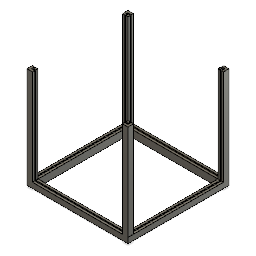
Bofy-top (Autodesk Fusion 360 design; units mm, degrees)
Autodesk Fusion 360 part; units mm, degrees
sketch "Sketch10" plane through (0, 0, 0) normal (0, 1, 0) x (1, 0, 0)
  line L0 (-70, -70) -> (100, -70)
  line L1 (100, -70) -> (100, 100)
  line L2 (100, 100) -> (-70, 100)
  line L3 (-70, 100) -> (-70, -70)
  dimension "d21" = 170
  dimension "d22" = 170
  constraint horizontal L0
  constraint vertical L1
  constraint horizontal L2
  constraint vertical L3
  measures "d21" distance of L0.start L0.end
  measures "d22" distance of L0.start L2.end
extrude "Extrude8" add sketch "Sketch10" along normal blind 8 makes body 1
sketch "Sketch11" plane through (0, 8, 0) normal (0, 1, 0) x (-1, 0, 0)
  line L0 (70, -100) -> (70, 70)
  line L1 (70, 70) -> (-100, 70)
  line L2 (-100, 70) -> (-100, -100)
  line L3 (-100, -100) -> (70, -100)
  line L4 (65, -95) -> (-95, -95)
  line L5 (-95, -95) -> (-95, 65)
  line L6 (-95, 65) -> (65, 65)
  line L7 (65, 65) -> (65, -95)
  constraint horizontal L4
  constraint vertical L5
  constraint horizontal L6
  constraint vertical L7
extrude "Extrude9" cut sketch "Sketch11" against normal blind 8 contours L4 L5 L6 L7 bodies 1
sketch "Sketch12" plane through (0, 8, 0) normal (0, 1, 0) x (-1, 0, 0)
  line L0 (-95, -95) -> (-95, 65)
  line L1 (-95, 65) -> (65, 65)
  line L2 (65, 65) -> (65, -95)
  line L3 (65, -95) -> (-95, -95)
  line L4 (70, -100) -> (70, 70)
  line L5 (70, 70) -> (-100, 70)
  line L6 (-100, 70) -> (-100, -100)
  line L7 (-100, -100) -> (70, -100)
  line L8 (75, -105) -> (-105, -105)
  line L9 (-105, -105) -> (-105, 75)
  line L10 (-105, 75) -> (75, 75)
  line L11 (75, 75) -> (75, -105)
  constraint horizontal L8
  constraint vertical L9
  constraint horizontal L10
  constraint vertical L11
extrude "Extrude10" add sketch "Sketch12" against normal blind 5 separate body contours L8 L9 L10 L11 makes body 2
sketch "Sketch15" plane through (0, 0, 0) normal (0, 1, 0) x (1, 0, 0)
sketch "Sketch16" plane through (0, 8, 0) normal (0, 1, 0) x (-1, 0, 0)
  line L0 (70, -100) -> (-100, -100)
  line L1 (-100, -100) -> (-100, 70)
  line L2 (-100, 70) -> (70, 70)
  line L3 (70, 70) -> (70, -100)
  line L4 (75, 75) -> (-105, 75)
  line L5 (-105, 75) -> (-105, -105)
  line L6 (-105, -105) -> (75, -105)
  line L7 (75, -105) -> (75, 75)
  line L8 (75, -105) -> (-105, -105)
  line L9 (-105, -105) -> (-105, 75)
  line L10 (-105, 75) -> (75, 75)
  line L11 (75, 75) -> (75, -105)
  constraint horizontal L8
  constraint vertical L9
  constraint horizontal L10
  constraint vertical L11
  constraint coincident L4.end L5.start
  constraint coincident L6.end L7.start
extrude "Extrude11" add sketch "Sketch16" along normal blind 5 bodies 2 1
sketch "Sketch17" plane through (0, 0, -100) normal (0, 0, 1) x (1, 0, 0)
  line L0 (-70, 8) -> (100, 8)
  line L1 (100, 8) -> (100, 13)
  line L2 (100, 13) -> (-70, 13)
  line L3 (-70, 13) -> (-70, 8)
sketch "Sketch18" plane through (0, 13, 0) normal (0, 1, 0) x (-1, 0, 0)
  line L0 (-100, 70) -> (70, 70)
  line L1 (70, 70) -> (70, -100)
  line L2 (70, -100) -> (-100, -100)
  line L3 (-100, -100) -> (-100, 70)
  line L4 (75, 75) -> (-105, 75)
  line L5 (-105, 75) -> (-105, -105)
  line L6 (-105, -105) -> (75, -105)
  line L7 (75, -105) -> (75, 75)
  line L8 (71, -101) -> (-101, -101)
  line L9 (-101, -101) -> (-101, 71)
  line L10 (-101, 71) -> (71, 71)
  line L11 (71, 71) -> (71, -101)
  dimension "d31" = 172
  dimension "d32" = 172
  constraint horizontal L8
  constraint vertical L9
  constraint horizontal L10
  constraint vertical L11
  measures "d31" distance of L8.start L8.end
  measures "d32" distance of L8.start L10.end
extrude "Extrude12" cut sketch "Sketch18" against normal blind 5 contours L8 L9 L10 L11 bodies 2
sketch "Sketch19" plane through (0, 8, 0) normal (0, 1, 0) x (-1, 0, 0)
  line L0 (71, 71) -> (-101, 71)
  line L1 (-101, 71) -> (-101, -101)
  line L2 (-101, -101) -> (71, -101)
  line L3 (71, -101) -> (71, 71)
  line L4 (-95, -95) -> (-95, 65)
  line L5 (-95, 65) -> (65, 65)
  line L6 (65, 65) -> (65, -95)
  line L7 (65, -95) -> (-95, -95)
  line L8 (69, -99) -> (-99, -99)
  line L9 (-99, -99) -> (-99, 69)
  line L10 (-99, 69) -> (69, 69)
  line L11 (69, 69) -> (69, -99)
  dimension "d35" = 168
  dimension "d36" = 168
  constraint horizontal L8
  constraint vertical L9
  constraint horizontal L10
  constraint vertical L11
  measures "d35" distance of L8.start L10.end
  measures "d36" distance of L8.start L8.end
extrude "Extrude13" add sketch "Sketch19" along normal blind 5 contours L8 L9 L10 L11 bodies 2
sketch "Sketch20" plane through (0, 13, 0) normal (0, 1, 0) x (-1, 0, 0)
  line L0 (-101, -101) -> (-101, 71)
  line L1 (-101, 71) -> (71, 71)
  line L2 (71, 71) -> (71, -101)
  line L3 (71, -101) -> (-101, -101)
  line L4 (75, 75) -> (-105, 75)
  line L5 (-105, 75) -> (-105, -105)
  line L6 (-105, -105) -> (75, -105)
  line L7 (75, -105) -> (75, 75)
  line L8 (75, -105) -> (65, -105)
  line L9 (65, -105) -> (65, -95)
  line L10 (65, -95) -> (75, -95)
  line L11 (75, -95) -> (75, -105)
  point P0 (65, -95)
  constraint horizontal L8
  constraint vertical L9
  constraint horizontal L10
  constraint vertical L11
  constraint coincident P0 L9.end
  constraint coincident L6.end L7.start
extrude "Extrude14" add sketch "Sketch20" along normal blind 170 contours L2 L3 L9 L10 | L2 L3 L6 L7 L8 L9 L10 L11 bodies 2
sketch "Sketch21" plane through (0, 183, 0) normal (0, 1, 0) x (-1, 0, 0)
  line L0 (75, -95) -> (65, -95)
  line L1 (65, -95) -> (65, -105)
  line L2 (65, -105) -> (75, -105)
  line L3 (75, -105) -> (75, -95)
  line L4 (65, -101) -> (71, -101)
  line L5 (71, -101) -> (71, -95)
  line L6 (69, -95) -> (69, -99)
  line L7 (69, -99) -> (65, -99)
  point P0 (65, -101)
  point P1 (71, -101)
  point P2 (71, -95)
  point P3 (69, -95)
  point P4 (69, -99)
  point P5 (65, -99)
  constraint coincident P0 L4.start
  constraint coincident P1 L4.end
  constraint coincident P2 L5.end
  constraint coincident P3 L6.start
  constraint coincident P4 L6.end
  constraint coincident P5 L7.end
extrude "Extrude15" cut sketch "Sketch21" against normal blind 170 contours L0 L1 L4 L5 L6 L7 bodies 2
sketch "Sketch22" plane through (0, 13, 0) normal (0, 1, 0) x (-1, 0, 0)
  line L0 (65, -105) -> (65, -101)
  line L1 (65, -101) -> (-101, -101)
  line L2 (-101, -101) -> (-101, 71)
  line L3 (-101, 71) -> (71, 71)
  line L4 (71, 71) -> (71, -95)
  line L5 (71, -95) -> (75, -95)
  line L6 (75, -95) -> (75, 75)
  line L7 (75, 75) -> (-105, 75)
  line L8 (-105, 75) -> (-105, -105)
  line L9 (-105, -105) -> (65, -105)
  line L10 (65, 65) -> (69, 65)
  line L11 (69, 65) -> (69, 69)
  line L12 (69, 69) -> (65, 69)
  line L13 (65, 69) -> (65, 65)
  line L14 (75, 64.9755) -> (75, 75)
  line L15 (75, 75) -> (65, 75)
  line L16 (65, 75) -> (65, 71)
  line L17 (65, 71) -> (71, 71)
  line L18 (71, 71) -> (71, 65)
  line L19 (71, 65) -> (75, 64.9755)
  point P0 (65, 65)
  point P1 (69, 69)
  constraint horizontal L10
  constraint vertical L11
  constraint horizontal L12
  constraint vertical L13
  constraint coincident P1 L11.end
  constraint coincident P0 L10.start
  constraint coincident L6 L14.start
  constraint coincident L6.end L7.start
  constraint perpendicular L7 L14
  constraint coincident L7 L15.end
  constraint perpendicular L6 L15
  constraint perpendicular L7 L16
  constraint coincident L3.end L4.start
  constraint coincident L4 L18.end
  constraint perpendicular L3 L18
extrude "Extrude16" add sketch "Sketch22" along normal blind 170 contours L3 L4 L6 L7 L14 L15 L16 L17 L18 L19 | L10 L11 L12 L13 bodies 2
sketch "Sketch23" plane through (0, 13, 0) normal (0, 1, 0) x (-1, 0, 0)
  line L0 (65, 65) -> (65, 69)
  line L1 (65, 69) -> (-99, 69)
  line L2 (-99, 69) -> (-99, -99)
  line L3 (-99, -99) -> (65, -99)
  line L4 (65, -99) -> (65, -95)
  line L5 (65, -95) -> (-95, -95)
  line L6 (-95, -95) -> (-95, 65)
  line L7 (-95, 65) -> (65, 65)
  line L8 (-95, 65) -> (-99, 65)
  line L9 (-99, 65) -> (-99, 69)
  line L10 (-99, 69) -> (-95, 69)
  line L11 (-95, 69) -> (-95, 65)
  constraint horizontal L8
  constraint vertical L9
  constraint horizontal L10
  constraint vertical L11
  constraint coincident L1.end L2.start
  constraint coincident L6.end L7.start
sketch "Sketch24" plane through (0, 13, 0) normal (0, 1, 0) x (-1, 0, 0)
  line L0 (65, 71) -> (65, 75)
  line L1 (65, 75) -> (-105, 75)
  line L2 (-105, 75) -> (-105, -105)
  line L3 (-105, -105) -> (65, -105)
  line L4 (65, -105) -> (65, -101)
  line L5 (65, -101) -> (-101, -101)
  line L6 (-101, -101) -> (-101, 71)
  line L7 (-101, 71) -> (65, 71)
  line L8 (-101, 65) -> (-105, 65)
  line L9 (-105, 65) -> (-105, 75)
  line L10 (-105, 75) -> (-95, 75)
  line L11 (-95, 75) -> (-95, 71)
  line L12 (-95, 71) -> (-101, 71)
  line L13 (-101, 71) -> (-101, 65)
  constraint coincident L6 L8.start
  constraint coincident L2 L8.end
  constraint coincident L1.end L2.start
  constraint coincident L1 L10.end
  constraint perpendicular L2 L10
  constraint coincident L7 L11.end
  constraint coincident L6.end L7.start
extrude "Extrude17" add sketch "Sketch23" sketch "Sketch24" along normal blind 170 contours L1 L2 L8 L9 L10 L11 of sketch 2 contours L1 L2 L6 L7 L8 L9 L10 L11 L12 L13 bodies 2
sketch "Sketch25" plane through (0, 13, 0) normal (0, 1, 0) x (-1, 0, 0)
  line L0 (-95, 65) -> (-99, 65)
  line L1 (-99, 65) -> (-99, -99)
  line L2 (-99, -99) -> (65, -99)
  line L3 (65, -99) -> (65, -95)
  line L4 (65, -95) -> (-95, -95)
  line L5 (-95, -95) -> (-95, 65)
  line L6 (-95, -95) -> (-99, -95)
  line L7 (-99, -95) -> (-99, -99)
  line L8 (-99, -99) -> (-95, -99)
  line L9 (-95, -99) -> (-95, -95)
  line L10 (65, -101) -> (-101, -101)
  line L11 (-105, -105) -> (65, -105)
  line L12 (-95, -101) -> (-95, -105)
  line L13 (-95, -105) -> (-105, -105)
  line L14 (-105, -105) -> (-105, 75)
  line L15 (-105, -105) -> (-105, -95)
  line L16 (-105, -95) -> (-101, -95)
  line L17 (-101, -95) -> (-101, -101)
  line L18 (-101, -101) -> (-95, -101)
  constraint horizontal L6
  constraint vertical L7
  constraint horizontal L8
  constraint vertical L9
  constraint coincident L1.end L2.start
  constraint coincident L4.end L5.start
  constraint coincident L10 L12.start
  constraint coincident L11 L12.end
  constraint perpendicular L2 L12
  constraint coincident L11.start L13.end
  constraint coincident L14 L15.end
  constraint perpendicular L14 L16
  constraint coincident L10.end L17.end
extrude "Extrude18" add sketch "Sketch25" along normal blind 170 contours L1 L2 L6 L7 L8 L9 | L10 L11 L12 L13 L14 L15 L16 L17 L18 bodies 2
sketch "Sketch13" plane through (105, 0, 0) normal (1, 0, 0) x (0, 0, -1)
  line L0 (-75, 8) -> (105, 8)
  line L1 (105, 8) -> (105, 13)
  line L2 (105, 13) -> (-75, 13)
  line L3 (-75, 13) -> (-75, 8)
sketch "Sketch14" plane through (0, 8, 0) normal (0, 1, 0) x (-1, 0, 0)
  line L0 (-95, -95) -> (-95, 65)
  line L1 (-95, 65) -> (65, 65)
  line L2 (65, 65) -> (65, -95)
  line L3 (65, -95) -> (-95, -95)
  line L4 (70, -100) -> (70, 70)
  line L5 (70, 70) -> (-100, 70)
  line L6 (-100, 70) -> (-100, -100)
  line L7 (-100, -100) -> (70, -100)
extrude "Extrude1" [suppressed]
sketch "Sketch2" plane through (0, 0, 0) normal (0, -1, 0) x (1, 0, 0)
  line L0 (94.1899, 85.4163) -> (-85.8101, 85.4163)
  line L1 (-85.8101, 85.4163) -> (-85.8101, -94.5837)
  line L2 (-85.8101, -94.5837) -> (94.1899, -94.5837)
  line L3 (94.1899, -94.5837) -> (94.1899, 85.4163)
